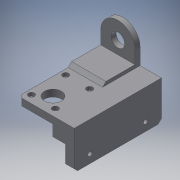
# Autodesk Inventor part: frame
Saved by Autodesk Inventor 2017 (Build 210142000, 142)
## iProperties
Created: 2018-01-02
Part Number: frame
Material: Generic
Document SubType Name: Modeling
Designer: RLanting
Density: 1 g/cm^3
Appearance: Default
Author: RLanting
Autodesk Inventor part; units mm, degrees
ref_plane "YZ Plane" through (0, 0, 0) normal (1, 0, 0) x (0, 1, 0)
ref_plane "XZ Plane" through (0, 0, 0) normal (0, 1, 0) x (-1, 0, 0)
ref_plane "XY Plane" through (0, 0, 0) normal (0, 0, 1) x (1, 0, 0)
sketch "Sketch1" plane through (0, 0, 0) normal (0, 0, 1) x (1, 0, 0)
  line L0 (14, -20) -> (-14, -20) construction
  line L1 (-14, -20) -> (-14, 20) construction
  line L2 (-14, 20) -> (14, 20) construction
  line L3 (14, 20) -> (14, -20) construction
  line L4 (14, -20) -> (-14, 20) construction
  line L5 (-14, -20) -> (14, 20) construction
  circle A0 centre (-14, 20) radius 2.25
  circle A1 centre (14, 20) radius 2.25
  circle A2 centre (14, -20) radius 2.25
  circle A3 centre (-14, -20) radius 2.25
  line L6 (0, 0) -> (0, -8.85) construction
  circle A4 centre (0, -8.85) radius 10
  line L7 (20.06, -29.05) -> (-20.06, -29.05)
  line L8 (-20.06, -29.05) -> (-20.06, 29.05)
  line L9 (-20.06, 29.05) -> (20.06, 29.05)
  line L10 (20.06, 29.05) -> (20.06, -29.05)
  line L11 (20.06, -29.05) -> (-20.06, 29.05) construction
  line L12 (-20.06, -29.05) -> (20.06, 29.05) construction
  dimension "d0" = 28
  dimension "d1" = 40
  dimension "d2" = 20
  dimension "d3" = 4.5
  dimension "d4" = 58.1
  dimension "d5" = 40.12
  dimension "d6" = 37.9
  constraints: 26 end point, 5 centre point, 5 coincident, 4 midpoint, 4 parallel, 3 equal radius, 2 horizontal, 2 perpendicular, 1 vertical
  measures "d0" distance of L1.end L2.end
  measures "d1" distance of L0.end L1.end
  measures "d2" diameter of A4
  measures "d3" diameter of A0
  measures "d4" distance of L9.end L7.start
  measures "d5" distance of L8.end L9.end
  measures "d6" distance from line of L6.end L9
extrude "Extrusion1" add sketch "Sketch1" along normal blind 8
sketch "Sketch2" plane through (0, 0, 8) normal (0, 0, 1) x (1, 0, 0)
  circle A0 centre (0, -8.85) radius 10 construction
  circle A1 centre (-14, -20) radius 2.25 construction
  circle A2 centre (14, -20) radius 2.25 construction
  circle A3 centre (14, 20) radius 2.25 construction
  circle A4 centre (-14, 20) radius 2.25 construction
  line L0 (-20.06, -29.05) -> (20.06, -29.05) construction
  line L1 (20.06, -29.05) -> (20.06, 29.05) construction
  line L2 (20.06, 29.05) -> (-20.06, 29.05) construction
  line L3 (-20.06, 29.05) -> (-20.06, -29.05) construction
  circle A5 centre (14, -20) radius 3.5
  circle A6 centre (-14, -20) radius 3.5
  circle A7 centre (14, 20) radius 3.5
  circle A8 centre (-14, 20) radius 3.5
  point P0 (0, 0)
  dimension "d9" = 7
  constraints: 4 centre point, 4 coincident, 3 equal radius
  measures "d9" diameter of A5
extrude "Extrusion2" cut sketch "Sketch2" against normal blind 4
sketch "Sketch3" plane through (-20.06, 29.05, 0) normal (0, 1, 0) x (1, 0, 0)
  line L0 (40.12, 0) -> (0, 0)
  line L1 (0, 0) -> (0, -12)
  line L2 (0, -12) -> (40.12, -12)
  line L3 (40.12, -12) -> (40.12, 0)
  circle A0 centre (20.06, 19.7) radius 15.5 construction
  line L4 (40.12, 0) -> (33.3508, 11.7247)
  line L5 (0, 0) -> (6.7692, 11.7247)
  arc A1 (6.7692, 11.7247) -> (33.3508, 11.7247) centre (20.06, 19.7) ccw
  line L6 (40.12, 0) -> (0, 0) projected
  line L7 (40.12, 0) -> (0, 0)
  point P0 (20.06, 0)
  dimension "d12" = 12
  dimension "d19" = 60
  constraints: 14 end point, 4 equal length, 4 point on circle, 3 coincident, 1 centre point, 1 horizontal, 1 perpendicular
  measures "d12" distance of L0.end L1.end
  measures "d19" angle of L0 L4
extrude "Extrusion3" add sketch "Sketch3" along normal blind 40
sketch "Sketch4" plane through (-20.06, 69.05, 0) normal (0, 1, 0) x (1, 0, 0)
  line L0 (20.06, 0) -> (20.06, -27) construction
  circle A0 centre (20.06, -27) radius 8
  line L1 (20.06, -27) -> (20.06, 0) construction
  line L2 (40.12, 0) -> (0, 0) projected
  line L3 (40.12, -27) -> (40.12, 0)
  line L4 (0, 0) -> (0, -27)
  arc A1 (0, -27) -> (40.12, -27) centre (20.06, -27) ccw
  arc A2 (40.12, 0) -> (0, 0) centre (20.06, 0) ccw construction
  line L5 (40.12, 0) -> (40.12, -8) projected
  line L6 (40.12, 0) -> (0, 0)
  line L7 (0, 0) -> (40.12, 0)
  line L8 (40.12, 0) -> (33.3508, 11.7247) projected
  arc A3 (6.7692, 11.7247) -> (33.3508, 11.7247) centre (20.06, 19.7) ccw projected
  line L9 (6.7692, 11.7247) -> (0, 0) projected
  line L10 (0, 0) -> (0, -12) projected
  line L11 (0, -12) -> (40.12, -12) projected
  line L12 (40.12, -12) -> (40.12, 0) projected
  point P0 (20.06, -13.5)
  dimension "d15" = 27
  dimension "d16" = 16
  constraints: 14 end point, 4 point on circle, 4 tangent, 3 centre point, 2 equal length, 1 coincident, 1 horizontal, 1 midpoint, 1 perpendicular, 1 point on line, 1 vertical
  measures "d15" distance of L0.start L0.end
  measures "d16" diameter of A0
extrude "Extrusion4" add sketch "Sketch4" along normal blind 6
sketch "Sketch5" plane through (-20.06, -29.05, 0) normal (0, -1, 0) x (1, 0, 0)
  line L0 (40.12, 0) -> (40.12, 8) projected
  line L1 (40.12, 8) -> (65.12, 8)
  line L2 (65.12, 8) -> (65.12, -17)
  line L3 (65.12, -17) -> (40.12, -17)
  line L4 (40.12, -17) -> (40.12, 8)
  line L5 (40.12, 0) -> (33.3508, -11.7247) projected
  line L6 (33.3508, -11.7247) -> (40.12, -17)
  line L7 (40.12, 27) -> (40.12, 0) projected
  line L8 (40.12, -17) -> (40.12, 0)
  point P0 (20.06, 0)
  dimension "d20" = 25
  dimension "d21" = 25
  constraints: 12 end point, 2 parallel, 1 horizontal, 1 perpendicular, 1 vertical
  measures "d20" distance of L1.end L2.end
  measures "d21" distance of L2.end L3.end
extrude "Extrusion5" add sketch "Sketch5" against normal up to surface (58.1 mm away) contours L0 L1 L2 L3 L4
sketch "Sketch6" plane through (20.06, 29.05, -17) normal (0, 1, 0) x (1, 0, 0)
  line L0 (25, 0) -> (0, 0) projected
  line L1 (0, 0) -> (0, -17) projected
  line L2 (0, -25) -> (0, -17) projected
  line L3 (0, -25) -> (25, -25) projected
  line L4 (25, -25) -> (25, 0) projected
  line L5 (0, -17) -> (-6.7692, -5.2753) projected
  line L6 (25, 0) -> (0, 0) projected
  line L7 (0, 0) -> (-6.7692, -5.2753)
  line L8 (0, 0) -> (0, -17) projected
  line L9 (0, -17) -> (0, 0)
  point P0 (-20.06, -17)
  constraints: 4 end point, 1 collinear
extrude "Extrusion6" add sketch "Sketch6" along normal up to surface (46 mm away)
sketch "Sketch7" plane through (45.06, -29.05, 8) normal (1, 0, 0) x (0, 0, -1)
  line L0 (25, 104.1) -> (0, 104.1) projected
  line L1 (25, 0) -> (25, 104.1) projected
  line L2 (25, 104.1) -> (25, 0)
  line L3 (25, 0) -> (45, 0)
  line L4 (45, 0) -> (45, 104.1)
  line L5 (45, 104.1) -> (25, 104.1)
  point P0 (8, 29.05)
  dimension "d26" = 20
  constraints: 8 end point, 2 parallel, 1 perpendicular, 1 vertical
  measures "d26" distance of L4.end L0.start
extrude "Extrusion7" add sketch "Sketch7" against normal blind 10
sketch "Sketch8" plane through (35.06, -29.05, 8) normal (-1, 0, 0) x (0, 0, 1)
  line L0 (-25, 104.1) -> (-25, 0) projected
  line L1 (-25, 104.1) -> (-45, 104.1) projected
  line L2 (-45, 104.1) -> (-45, 0) projected
  line L3 (-45, 0) -> (-25, 0) projected
  line L4 (-45, 104.1) -> (-45, 0) projected
  line L5 (-45, 52.05) -> (-25, 52.05) construction
  line L6 (-35, 84.55) -> (-35, 19.55) construction
  circle A0 centre (-35, 84.55) radius 2.5
  circle A1 centre (-35, 19.55) radius 2.5
  point P0 (-8, 29.05)
  point P1 (-35, 52.05)
  dimension "d29" = 65
  dimension "d30" = 5
  constraints: 4 end point, 4 midpoint, 2 centre point, 2 coincident, 1 equal radius, 1 vertical
  measures "d29" distance of L6.start L6.end
  measures "d30" diameter of A0
extrude "Extrusion8" cut sketch "Sketch8" against normal through all contours A0 | A1
chamfer "Chamfer1" distance 4 angle 45 5 edges at (40.06, 75.05, -37) (40.06, -29.05, -37) (27.56, -29.05, -17) (-20.06, -29.05, 4) (0, 29.05, 12)
sketch "Sketch9" plane through (-20.06, 75.05, 0) normal (0, 1, 0) x (1, 0, 0)
  circle A0 centre (20.06, 19.7) radius 15.5 construction
  circle A1 centre (20.06, 19.7) radius 16.5
  point P0 (20.06, 0)
  dimension "d36" = 1
  constraints: 1 centre point, 1 coincident
  measures "d36" radial gap between concentric circles of A0 A1
extrude "Extrusion9" cut sketch "Sketch9" against normal up to surface (46 mm away)
body "Solid1"
